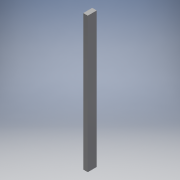
# Autodesk Inventor part: base
Saved by Autodesk Inventor 2017 (Build 210142000, 142)
## iProperties
Created: 2022-03-14
Part Number: base
Material: Stahl
Document SubType Name: Modeling
Designer: 10154704
Density: 7.85 g/cm^3
Appearance: Stahl
Author: 10154704
Autodesk Inventor part; units mm, degrees
ref_plane "YZ Plane" through (0, 0, 0) normal (1, 0, 0) x (0, 1, 0)
ref_plane "XZ Plane" through (0, 0, 0) normal (0, 1, 0) x (-1, 0, 0)
ref_plane "XY Plane" through (0, 0, 0) normal (0, 0, 1) x (1, 0, 0)
sketch "Skizze1" plane through (0, 0, 0) normal (0, 0, 1) x (1, 0, 0)
  line L0 (0, 0) -> (10, 0)
  line L1 (10, 0) -> (10, 20)
  line L2 (10, 20) -> (0, 20)
  line L3 (0, 20) -> (0, 0)
  dimension "d2" = 10
  dimension "d3" = 20
  constraints: 8 end point, 2 parallel, 1 horizontal, 1 perpendicular
  measures "d2" distance between parallel lines of L1 L3
  measures "d3" distance between parallel lines of L0 L2
extrude "Extrusion1" add sketch "Skizze1" along normal mid plane 300
